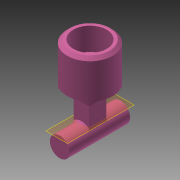
# Autodesk Inventor part: wrist-forearm
Saved by Autodesk Inventor 2016 (Build 200138000, 138)
## iProperties
Created: 2015-10-08
Part Number: wrist-forearm
Material: Generic
Document SubType Name: Modeling
Designer: eedoga
Density: 1 g/cm^3
Appearance: Pink
Author: eedoga
Autodesk Inventor part; units mm, degrees
ref_plane "YZ Plane" through (0, 0, 0) normal (1, 0, 0) x (0, 1, 0)
sketch "Sketch1" plane through (0, 0, 0) normal (0, 0, 1) x (1, 0, 0)
  arc A0 (6.35, 20.6311) -> (19.05, 20.6311) centre (12.7, 12.7) ccw projected
  circle A1 centre (12.7, 12.7) radius 8.255
  point P0 (0, 0)
  dimension "d0" = 16.51
  constraints: 1 centre point, 1 coincident
  measures "d0" diameter of A1
extrude "Extrusion1" add sketch "Sketch1" against normal blind 50.8
ref_plane "Work Plane1" through (12.7, 20.955, 0) normal (0, 1, 0) x (-1, 0, 0)
sketch "Sketch2" plane through (12.7, 20.955, 0) normal (0, 1, 0) x (-1, 0, 0)
  line L0 (6.35, -15.875) -> (12.7, -15.875) projected
  line L1 (-12.7, -15.875) -> (-6.35, -15.875) projected
  line L2 (-6.35, -34.925) -> (-12.7, -34.925) projected
  line L3 (12.7, -34.925) -> (6.35, -34.925) projected
  line L4 (-8.255, -50.8) -> (8.255, -50.8) projected
  line L5 (-8.255, 0) -> (8.255, 0) projected
  line L6 (-6.4396, -15.875) -> (-6.4396, -34.925)
  line L7 (-6.4396, -34.925) -> (-6.4396, -25.4)
  line L8 (-6.4396, -34.925) -> (-6.4396, -30.1625)
  line L9 (6.4396, -15.875) -> (6.4396, -34.925)
  line L10 (6.4396, -25.4) -> (6.4396, -15.875)
  line L11 (6.4396, -20.6375) -> (6.4396, -15.875)
  line L12 (-6.4396, -32.5438) -> (6.4396, -32.5438)
  line L13 (6.4396, -32.5438) -> (6.4396, -18.2563)
  line L14 (6.4396, -18.2563) -> (-6.4396, -18.2563)
  line L15 (-6.4396, -18.2563) -> (-6.4396, -32.5438)
  point P0 (12.7, 0)
  constraints: 20 end point, 6 midpoint, 4 point on line, 3 perpendicular, 2 collinear, 2 parallel, 1 horizontal
extrude "Extrusion2" add sketch "Sketch2" along normal blind 25.4 and the other way blind 8.255
chamfer "Chamfer1" distance 1.27 angle 45 2 edges at (12.7, 20.955, -18.2563) (12.7, 20.955, -32.5438)
sketch "Sketch3" plane through (12.7, 46.355, 0) normal (0, 1, 0) x (1, 0, 0)
  line L0 (6.4396, 32.5438) -> (-6.4396, 32.5438) projected
  line L1 (-6.4396, 32.5438) -> (-6.4396, 18.2563) projected
  line L2 (-6.4396, 18.2563) -> (6.4396, 18.2563) projected
  line L3 (6.4396, 18.2563) -> (6.4396, 32.5438) projected
  line L4 (-6.4396, 18.2563) -> (6.4396, 32.5438)
  line L5 (6.4396, 18.2563) -> (-6.4396, 32.5438)
  circle A0 centre (0, 25.4) radius 19.05
  circle A1 centre (0, 25.4) radius 13.97
  point P0 (-12.7, 0)
  dimension "d11" = 38.1
  dimension "d12" = 27.94
  constraints: 4 end point, 2 centre point, 1 coincident, 1 midpoint
  measures "d11" diameter of A0
  measures "d12" diameter of A1
extrude "Extrusion3" add sketch "Sketch3" along normal blind 12.7 contours L4 L5 L0 | L3 L5 L4 | L5 L4 L1 | L2 L4 L5 | A1
extrude "Extrusion4" add sketch "Sketch3" along normal blind 31.75 contours A0
chamfer "Chamfer2" distance 10.16 angle 45 4 edges at (6.2604, 46.355, -25.4) (12.7, 46.355, -18.2563) (19.1396, 46.355, -25.4) (12.7, 46.355, -32.5438)
chamfer "Chamfer3" distance 2.54 angle 45 1 edges at (-6.35, 78.105, -25.4)
ref_plane "Work Plane2" through (4.445, 12.7, 0) normal (1, 0, 0) x (0, 1, 0)
sketch "Sketch4" plane through (19.1396, 17.8649, -16.9863) normal (1, 0, 0) x (0, 0, -1)
  line L0 (1.27, 18.3301) -> (15.5575, 18.3301) projected
  line L1 (1.27, 1.8534) -> (1.27, 18.3301) projected
  line L2 (16.8275, 0) -> (0, 0) projected
  line L3 (15.5575, 18.3301) -> (15.5575, 1.8534) projected
  line L4 (1.27, 1.8534) -> (15.5575, 1.8534)
  line L5 (8.4138, 1.8534) -> (8.4138, 4.3934)
  circle A0 centre (8.4138, 4.3934) radius 1.5875
  point P0 (-16.9863, -17.8649)
  dimension "d23" = 2.54
  dimension "d24" = 3.175
  constraints: 4 end point, 2 perpendicular, 1 centre point, 1 coincident, 1 midpoint, 2 other
  measures "d23" distance of L5.start L5.end
  measures "d24" diameter of A0
ref_plane "Work Plane3" through (19.1396, 17.8649, 0) normal (0.8660254, 0.5, 0) x (0, 0, 1)
sketch "Sketch5" plane through (19.1396, 17.8649, 0) normal (0.8660254, 0.5, 0) x (0, 0, 1)
  circle A0 centre (-25.4, -4.7625) radius 1.5875
  point P0 (0, 5.9017)
  dimension "d26" = 3.175
  constraints: 1 centre point
  measures "d26" diameter of A0
extrude "Extrusion5" cut sketch "Sketch5" along normal blind 12.7 and the other way blind 2.54
ref_plane "Work Plane4" through (12.7, 46.355, -6.35) normal (0, 0, 1) x (1, 0, 0)
sketch "Sketch6" plane through (12.7, 46.355, -6.35) normal (0, 0, 1) x (1, 0, 0)
  line L0 (16.5996, 0) -> (16.5996, 0) projected
  line L1 (16.5996, 0) -> (13.1137, -3.4859) projected
  arc A0 (13.1137, -3.4859) -> (7.9676, 0) centre (0, -17.3038) ccw projected
  line L2 (-7.9676, 0) -> (7.9676, 0) projected
  arc A1 (-7.9676, 0) -> (-13.1137, -3.4859) centre (0, -17.3038) ccw projected
  line L3 (-13.1137, -3.4859) -> (-16.5996, 0) projected
  line L4 (-16.5996, 0) -> (-16.5996, 0) projected
  line L5 (-16.5996, 0) -> (-13.1137, -3.4859) projected
  arc A2 (-7.9676, 0) -> (-13.1137, -3.4859) centre (0, -17.3038) ccw projected
  line L6 (7.9676, 0) -> (-7.9676, 0) projected
  arc A3 (13.1137, -3.4859) -> (7.9676, 0) centre (0, -17.3038) ccw projected
  line L7 (13.1137, -3.4859) -> (16.5996, 0) projected
  line L8 (19.05, 29.21) -> (-19.05, 29.21) projected
  line L9 (-19.05, 0) -> (-19.05, 29.21) projected
  line L10 (19.05, 0) -> (19.05, 29.21) projected
  line L11 (-19.05, 17.4625) -> (19.05, 17.4625)
  circle A4 centre (0, 17.4625) radius 1.5875
  point P0 (-12.7, -46.355)
  dimension "d31" = 3.175
  constraints: 2 end point, 2 point on line, 1 centre point, 1 midpoint, 1 perpendicular
  measures "d31" diameter of A4
hole "Hole1" at (12.7, 63.8175, -6.35) direction (0, 0, -1) diameter 3.175 end through all
ref_plane "Work Plane5" through (-240.4986, 445.264, 133.3441) normal (-0.8660254, -0.5, 0) x (-0.0199098, 0.0344847, -0.9992069)
sketch "Sketch7" plane through (-240.4986, 445.264, 133.3441) normal (-0.8660254, -0.5, 0) x (-0.0199098, 0.0344847, -0.9992069)
  circle A0 centre (25.4, -6.35) radius 1.5875
  point P0 (113.0953, 510.7677)
  dimension "d39" = 3.175
  constraints: 1 centre point
  measures "d39" diameter of A0
extrude "Extrusion6" cut sketch "Sketch7" against normal blind 12.7
body "Solid1"
